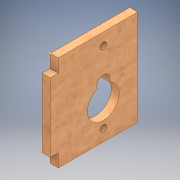
# Autodesk Inventor part: Podstawa-mocowanie serwa
Saved by Autodesk Inventor 2017 (Build 210142000, 142)
## iProperties
Created: 2017-05-18
Part Number: Podstawa-mocowanie serwa
Material: Drewno (wiśnia)
Document SubType Name: Modeling
Designer: Damian
Density: 0.63 g/cm^3
Appearance: Wiśnia — naturalna — niski połysk
Author: Damian
Autodesk Inventor part; units mm, degrees
ref_plane "YZ Plane" through (0, 0, 0) normal (1, 0, 0) x (0, 1, 0)
ref_plane "XZ Plane" through (0, 0, 0) normal (0, 1, 0) x (-1, 0, 0)
ref_plane "XY Plane" through (0, 0, 0) normal (0, 0, 1) x (1, 0, 0)
sketch "Szkic1" plane through (0, 0, 0) normal (0, 1, 0) x (-1, 0, 0)
  point P0 (0, 0)
sketch "Szkic2" plane through (0, 0, 0) normal (1, 0, 0) x (0, 1, 0)
  point P0 (0, 0)
sketch "Szkic3" plane through (0, 0, 0) normal (1, 0, 0) x (0, 1, 0)
  line L0 (0, 0) -> (30, 0)
  line L1 (30, 0) -> (30, -36)
  line L2 (30, -36) -> (0, -36)
  line L3 (0, -5) -> (-3, -5)
  line L4 (-3, -5) -> (-3, -31)
  line L5 (-3, -31) -> (0, -31)
  line L6 (0, -36) -> (0, -31)
  line L7 (0, -5) -> (0, 0)
  arc A0 (14.6923, -17.4615) -> (19.3077, -17.4615) centre (17, -23) ccw
  arc A1 (19.3077, -17.4615) -> (14.6923, -17.4615) centre (17, -16.5) ccw
  circle A2 centre (17, -31.5) radius 1.25
  circle A3 centre (17, -4.5) radius 1.25
  dimension "d1" = 36
  dimension "d4" = 5
  dimension "d5" = 26
  dimension "d6" = 3
  dimension "d7" = 30
  dimension "d8" = 13
  dimension "d9" = 13
  dimension "d10" = 4.5
  dimension "d11" = 4.5
  dimension "d12" = 6.5
  dimension "d13" = 12
  dimension "d14" = 5
  dimension "d15" = 2.5
  dimension "d16" = 2.5
  constraints: 16 end point, 4 centre point, 4 coincident, 4 parallel, 4 point on circle, 2 horizontal, 2 perpendicular
  measures "d1" distance of L0.end L1.end
  measures "d4" distance between parallel lines of L0 L3
  measures "d5" distance of L3.end L4.end
  measures "d6" distance of L4.end L5.end
  measures "d7" distance of L1.end L2.end
  measures "d8" distance from line of L1 point (17, -23)
  measures "d9" distance from line of L2 point (17, -23)
  measures "d10" distance from line of L2 point (17, -31.5)
  measures "d11" distance from line of L0 point (17, -4.5)
  measures "d12" distance of point (17, -16.5) point (17, -23)
  measures "d13" diameter of A0
  measures "d14" diameter of A1
  measures "d15" diameter of A2
  measures "d16" diameter of A3
extrude "Wyciągnięcie proste1" add sketch "Szkic3" along normal blind 3
